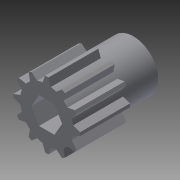
# Autodesk Inventor part: pinion
Saved by Autodesk Inventor 2015 SP1 (Build 190203100, 203)
## iProperties
Created: 2015-01-14
Part Number: pinion
Material: Generic
Document SubType Name: Modeling
Designer: Jarod
Density: 1 g/cm^3
Appearance: Default
Author: Jarod
Autodesk Inventor part; units mm, degrees
ref_plane "YZ Plane" through (0, 0, 0) normal (1, 0, 0) x (0, 1, 0)
ref_plane "XZ Plane" through (0, 0, 0) normal (0, 1, 0) x (-1, 0, 0)
ref_plane "XY Plane" through (0, 0, 0) normal (0, 0, 1) x (1, 0, 0)
sketch "Sketch1" plane through (0, 0, 0) normal (0, 0, 1) x (1, 0, 0)
  circle A0 centre (0, 0) radius 11.9062
  dimension "d0" = 23.8125
  constraints: 1 centre point, 1 coincident
  measures "d0" diameter of A0
extrude "Extrusion1" add sketch "Sketch1" along normal blind 41.275
sketch "Sketch2" plane through (0, 0, 41.275) normal (0, 0, 1) x (1, 0, 0)
  circle A0 centre (0, 0) radius 12.7
  dimension "d3" = 25.4
  constraints: 1 centre point, 1 coincident
  measures "d3" diameter of A0
extrude "Extrusion2" add sketch "Sketch2" against normal blind 23.8125
sketch "Sketch3" plane through (0, 0, 41.275) normal (0, 0, 1) x (1, 0, 0)
  line L0 (-3.6662, 6.35) -> (3.6662, 6.35)
  line L1 (3.6662, 6.35) -> (7.3323, 0)
  line L2 (7.3323, 0) -> (3.6662, -6.35)
  line L3 (3.6662, -6.35) -> (-3.6662, -6.35)
  line L4 (-3.6662, -6.35) -> (-7.3323, 0)
  line L5 (-7.3323, 0) -> (-3.6662, 6.35)
  point P0 (0, 0)
  dimension "d6" = 12.7
  dimension "d7" = 12.7
  dimension "d8" = 12.7
  dimension "d9" = 120
  dimension "d10" = 120
  dimension "d11" = 6.35
  dimension "d12" = 6.35
  dimension "d13" = 6.35
  constraints: 12 end point, 3 parallel, 1 horizontal
  measures "d6" distance between parallel lines of L3 L0
  measures "d7" distance between parallel lines of L4 L1
  measures "d8" distance between parallel lines of L2 L5
  measures "d9" angle of L0 L5
  measures "d10" angle of L1 L0
  measures "d11" distance from line of point (0, 0) L0
  measures "d12" distance from line of point (0, 0) L1
  measures "d13" distance from line of point (0, 0) L5
extrude "Extrusion3" cut sketch "Sketch3" against normal blind 50.8
sketch "Sketch4" plane through (0, 0, 41.275) normal (0, 0, 1) x (1, 0, 0)
  line L0 (-7.3323, 0) -> (-3.6662, 6.35) projected
  line L1 (-3.6662, 6.35) -> (3.6662, 6.35) projected
  line L2 (3.6662, 6.35) -> (7.3323, 0) projected
  line L3 (7.3323, 0) -> (3.6662, -6.35) projected
  line L4 (3.6662, -6.35) -> (-3.6662, -6.35) projected
  line L5 (-3.6662, -6.35) -> (-7.3323, 0) projected
  circle A0 centre (0, 0) radius 12.7 projected
  line L6 (0, 12.7) -> (0, 15.875) construction
  line L7 (0, 12.7) -> (3.175, 12.7) construction
  line L8 (0, 0) -> (1.9867, 12.5436) construction
  circle A1 centre (0, 0) radius 12.7 construction
  line L9 (0, 0) -> (12.7, 0) construction
  line L10 (0, 0) -> (-1.9867, 12.5436) construction
  line L11 (0, 0) -> (12.7, 0) construction
  line L12 (0, 15.875) -> (0.7937, 15.875) construction
  line L13 (0, 15.875) -> (0.7937, 15.875) construction
  line L14 (0, 15.875) -> (-0.7937, 15.875) construction
  line L15 (0, 15.875) -> (0.7937, 15.875) construction
  line L16 (-1.9867, 12.5436) -> (-0.7937, 15.875)
  line L17 (-0.7937, 15.875) -> (0.7937, 15.875)
  line L18 (0.7937, 15.875) -> (1.9867, 12.5436)
  line L19 (-1.9867, 12.5436) -> (1.9867, 12.5436)
  line L20 (-6.35, 10.9985) -> (-7.9375, 13.7482) construction
  line L21 (-6.35, 10.9985) -> (-3.6004, 12.586) construction
  line L22 (0, 0) -> (-4.5513, 11.8565) construction
  line L23 (0, 0) -> (-7.9924, 9.8698) construction
  line L24 (-7.9375, 13.7482) -> (-7.2501, 14.145) construction
  line L25 (-7.9375, 13.7482) -> (-7.2501, 14.145) construction
  line L26 (-7.9375, 13.7482) -> (-8.6249, 13.3513) construction
  line L27 (-7.9375, 13.7482) -> (-7.2501, 14.145) construction
  line L28 (-7.9924, 9.8698) -> (-8.6249, 13.3513)
  line L29 (-8.6249, 13.3513) -> (-7.2501, 14.145)
  line L30 (-7.2501, 14.145) -> (-4.5513, 11.8565)
  line L31 (-7.9924, 9.8698) -> (-4.5513, 11.8565)
  line L32 (-10.9985, 6.35) -> (-13.7482, 7.9375) construction
  line L33 (-10.9985, 6.35) -> (-9.411, 9.0996) construction
  line L34 (0, 0) -> (-9.8698, 7.9924) construction
  line L35 (0, 0) -> (-11.8565, 4.5513) construction
  line L36 (-13.7482, 7.9375) -> (-13.3513, 8.6249) construction
  line L37 (-13.7482, 7.9375) -> (-13.3513, 8.6249) construction
  line L38 (-13.7482, 7.9375) -> (-14.145, 7.2501) construction
  line L39 (-13.7482, 7.9375) -> (-13.3513, 8.6249) construction
  line L40 (-11.8565, 4.5513) -> (-14.145, 7.2501)
  line L41 (-14.145, 7.2501) -> (-13.3513, 8.6249)
  line L42 (-13.3513, 8.6249) -> (-9.8698, 7.9924)
  line L43 (-11.8565, 4.5513) -> (-9.8698, 7.9924)
  line L44 (-12.7, 0) -> (-15.875, 0) construction
  line L45 (-12.7, 0) -> (-12.7, 3.175) construction
  line L46 (0, 0) -> (-12.5436, 1.9867) construction
  line L47 (0, 0) -> (-12.5436, -1.9867) construction
  line L48 (-15.875, 0) -> (-15.875, 0.7938) construction
  line L49 (-15.875, 0) -> (-15.875, 0.7938) construction
  line L50 (-15.875, 0) -> (-15.875, -0.7937) construction
  line L51 (-15.875, 0) -> (-15.875, 0.7938) construction
  line L52 (-12.5436, -1.9867) -> (-15.875, -0.7937)
  line L53 (-15.875, -0.7937) -> (-15.875, 0.7938)
  line L54 (-15.875, 0.7938) -> (-12.5436, 1.9867)
  line L55 (-12.5436, -1.9867) -> (-12.5436, 1.9867)
  line L56 (-10.9985, -6.35) -> (-13.7482, -7.9375) construction
  line L57 (-10.9985, -6.35) -> (-12.586, -3.6004) construction
  line L58 (0, 0) -> (-11.8565, -4.5513) construction
  line L59 (0, 0) -> (-9.8698, -7.9924) construction
  line L60 (-13.7482, -7.9375) -> (-14.145, -7.2501) construction
  line L61 (-13.7482, -7.9375) -> (-14.145, -7.2501) construction
  line L62 (-13.7482, -7.9375) -> (-13.3513, -8.6249) construction
  line L63 (-13.7482, -7.9375) -> (-14.145, -7.2501) construction
  line L64 (-9.8698, -7.9924) -> (-13.3513, -8.6249)
  line L65 (-13.3513, -8.6249) -> (-14.145, -7.2501)
  line L66 (-14.145, -7.2501) -> (-11.8565, -4.5513)
  line L67 (-9.8698, -7.9924) -> (-11.8565, -4.5513)
  line L68 (-6.35, -10.9985) -> (-7.9375, -13.7482) construction
  line L69 (-6.35, -10.9985) -> (-9.0996, -9.411) construction
  line L70 (0, 0) -> (-7.9924, -9.8698) construction
  line L71 (0, 0) -> (-4.5513, -11.8565) construction
  line L72 (-7.9375, -13.7482) -> (-8.6249, -13.3513) construction
  line L73 (-7.9375, -13.7482) -> (-8.6249, -13.3513) construction
  line L74 (-7.9375, -13.7482) -> (-7.2501, -14.145) construction
  line L75 (-7.9375, -13.7482) -> (-8.6249, -13.3513) construction
  line L76 (-4.5513, -11.8565) -> (-7.2501, -14.145)
  line L77 (-7.2501, -14.145) -> (-8.6249, -13.3513)
  line L78 (-8.6249, -13.3513) -> (-7.9924, -9.8698)
  line L79 (-4.5513, -11.8565) -> (-7.9924, -9.8698)
  line L80 (0, -12.7) -> (0, -15.875) construction
  line L81 (0, -12.7) -> (-3.175, -12.7) construction
  line L82 (0, 0) -> (-1.9867, -12.5436) construction
  line L83 (0, 0) -> (1.9867, -12.5436) construction
  line L84 (0, -15.875) -> (-0.7938, -15.875) construction
  line L85 (0, -15.875) -> (-0.7938, -15.875) construction
  line L86 (0, -15.875) -> (0.7937, -15.875) construction
  line L87 (0, -15.875) -> (-0.7938, -15.875) construction
  line L88 (1.9867, -12.5436) -> (0.7937, -15.875)
  line L89 (0.7937, -15.875) -> (-0.7938, -15.875)
  line L90 (-0.7938, -15.875) -> (-1.9867, -12.5436)
  line L91 (1.9867, -12.5436) -> (-1.9867, -12.5436)
  line L92 (6.35, -10.9985) -> (7.9375, -13.7482) construction
  line L93 (6.35, -10.9985) -> (3.6004, -12.586) construction
  line L94 (0, 0) -> (4.5513, -11.8565) construction
  line L95 (0, 0) -> (7.9924, -9.8698) construction
  line L96 (7.9375, -13.7482) -> (7.2501, -14.145) construction
  line L97 (7.9375, -13.7482) -> (7.2501, -14.145) construction
  line L98 (7.9375, -13.7482) -> (8.6249, -13.3513) construction
  line L99 (7.9375, -13.7482) -> (7.2501, -14.145) construction
  line L100 (7.9924, -9.8698) -> (8.6249, -13.3513)
  line L101 (8.6249, -13.3513) -> (7.2501, -14.145)
  line L102 (7.2501, -14.145) -> (4.5513, -11.8565)
  line L103 (7.9924, -9.8698) -> (4.5513, -11.8565)
  line L104 (10.9985, -6.35) -> (13.7482, -7.9375) construction
  line L105 (10.9985, -6.35) -> (9.411, -9.0996) construction
  line L106 (0, 0) -> (9.8698, -7.9924) construction
  line L107 (0, 0) -> (11.8565, -4.5513) construction
  line L108 (13.7482, -7.9375) -> (13.3513, -8.6249) construction
  line L109 (13.7482, -7.9375) -> (13.3513, -8.6249) construction
  line L110 (13.7482, -7.9375) -> (14.145, -7.2501) construction
  line L111 (13.7482, -7.9375) -> (13.3513, -8.6249) construction
  line L112 (11.8565, -4.5513) -> (14.145, -7.2501)
  line L113 (14.145, -7.2501) -> (13.3513, -8.6249)
  line L114 (13.3513, -8.6249) -> (9.8698, -7.9924)
  line L115 (11.8565, -4.5513) -> (9.8698, -7.9924)
  line L116 (12.7, 0) -> (15.875, 0) construction
  line L117 (12.7, 0) -> (12.7, -3.175) construction
  line L118 (0, 0) -> (12.5436, -1.9867) construction
  line L119 (0, 0) -> (12.5436, 1.9867) construction
  line L120 (15.875, 0) -> (15.875, -0.7938) construction
  line L121 (15.875, 0) -> (15.875, -0.7938) construction
  line L122 (15.875, 0) -> (15.875, 0.7937) construction
  line L123 (15.875, 0) -> (15.875, -0.7938) construction
  line L124 (12.5436, 1.9867) -> (15.875, 0.7937)
  line L125 (15.875, 0.7937) -> (15.875, -0.7938)
  line L126 (15.875, -0.7938) -> (12.5436, -1.9867)
  line L127 (12.5436, 1.9867) -> (12.5436, -1.9867)
  line L128 (10.9985, 6.35) -> (13.7482, 7.9375) construction
  line L129 (10.9985, 6.35) -> (12.586, 3.6004) construction
  line L130 (0, 0) -> (11.8565, 4.5513) construction
  line L131 (0, 0) -> (9.8698, 7.9924) construction
  line L132 (13.7482, 7.9375) -> (14.145, 7.2501) construction
  line L133 (13.7482, 7.9375) -> (14.145, 7.2501) construction
  line L134 (13.7482, 7.9375) -> (13.3513, 8.6249) construction
  line L135 (13.7482, 7.9375) -> (14.145, 7.2501) construction
  line L136 (9.8698, 7.9924) -> (13.3513, 8.6249)
  line L137 (13.3513, 8.6249) -> (14.145, 7.2501)
  line L138 (14.145, 7.2501) -> (11.8565, 4.5513)
  line L139 (9.8698, 7.9924) -> (11.8565, 4.5513)
  line L140 (6.35, 10.9985) -> (7.9375, 13.7482) construction
  line L141 (6.35, 10.9985) -> (9.0996, 9.411) construction
  line L142 (0, 0) -> (7.9924, 9.8698) construction
  line L143 (0, 0) -> (4.5513, 11.8565) construction
  line L144 (7.9375, 13.7482) -> (8.6249, 13.3513) construction
  line L145 (7.9375, 13.7482) -> (8.6249, 13.3513) construction
  line L146 (7.9375, 13.7482) -> (7.2501, 14.145) construction
  line L147 (7.9375, 13.7482) -> (8.6249, 13.3513) construction
  line L148 (4.5513, 11.8565) -> (7.2501, 14.145)
  line L149 (7.2501, 14.145) -> (8.6249, 13.3513)
  line L150 (8.6249, 13.3513) -> (7.9924, 9.8698)
  line L151 (4.5513, 11.8565) -> (7.9924, 9.8698)
  dimension "d16" = 12.7
  dimension "d17" = 0
  dimension "d18" = 3.175
  dimension "d19" = 90
  dimension "d20" = 81
  dimension "d21" = 99
  dimension "d22" = 0.7937
  dimension "d23" = 0
  dimension "d24" = 0.7937
  dimension "d25" = 180
  dimension "d28" = 360
  constraints: 292 end point, 8 horizontal, 5 equal length, 2 point on circle, 1 vertical, 1 vertical alignment, 277 other
  measures "d16" distance of point (0, 0) L6.start
  measures "d17" horizontal distance of point (0, 0) L6.start
  measures "d18" distance of L6.start L6.end
  measures "d19" angle of L7 L6
  measures "d20" angle of L9 L8
  measures "d21" angle of L11 L10
  measures "d22" distance of L6.end L12.end
  measures "d23" distance between parallel lines of L12 L13
  measures "d24" distance of L6.end L14.end
  measures "d25" angle of L14 L15
extrude "Extrusion4" add sketch "Sketch4" against normal blind 23.8125 contours A0 L127 | A0 L124 L125 L126 | L139 A0 | A0 L136 L137 L138 | L112 L113 L114 A0 | A0 L115 | L151 A0 | A0 L148 L149 L150 | L100 L101 L102 A0 | A0 L103 | L19 A0 | A0 L16 L17 L18 | L88 L89 L90 A0 | A0 L91 | L31 A0 | A0 L28 L29 L30 | L76 L77 L78 A0 | A0 L79 | L43 A0 | A0 L40 L41 L42 | L64 L65 L66 A0 | A0 L67 | L55 A0 | A0 L52 L53 L54
body "Solid1"
